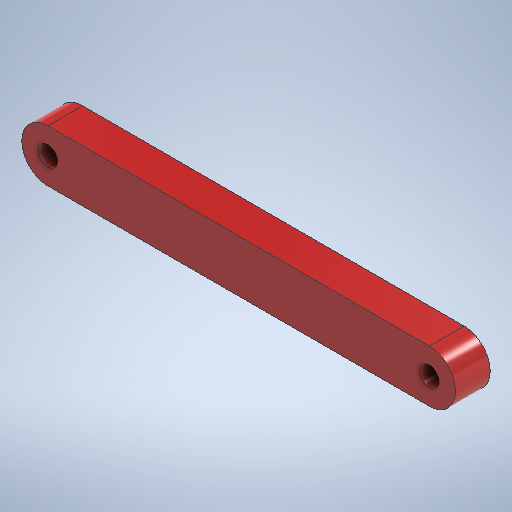
# Autodesk Inventor part: servostrap
Saved by Autodesk Inventor 2025.2 (Build 292293000, 293)
## iProperties
Created: 2025-04-02
Part Number: servostrap
Material: Generic
Document SubType Name: Modeling
Designer: m_kni
Density: 1 g/cm^3
Appearance: Default
Author: m_kni
## iProperties of the stored document servostrap_3DPrint.ipt
Created: 2025-04-02
Part Number: servostrap_3DPrint
Material: Generic
Document SubType Name: Modeling
Designer: m_kni
Density: 1 g/cm^3
Appearance: Default
Author: m_kni
Autodesk Inventor part; units mm, degrees
ref_plane "YZ Plane" through (0, 0, 0) normal (1, 0, 0) x (0, 1, 0)
ref_plane "XZ Plane" through (0, 0, 0) normal (0, 1, 0) x (-1, 0, 0)
ref_plane "XY Plane" through (0, 0, 0) normal (0, 0, 1) x (1, 0, 0)
sketch "Sketch1" plane through (0, 0, 0) normal (0, 0, 1) x (1, 0, 0)
  circle A0 centre (-21.9525, -0.0633) radius 1
  circle A1 centre (22.0475, -0.0633) radius 1
  circle A2 centre (-21.9525, -0.0633) radius 1.125
  circle A3 centre (22.0475, -0.0633) radius 1.125
  circle A4 centre (-21.9525, -0.0633) radius 3
  circle A5 centre (22.0475, -0.0633) radius 3
  line L0 (-21.9525, 2.9367) -> (22.0475, 2.9367)
  line L1 (-21.9525, -3.0633) -> (22.0475, -3.0633)
  point P0 (0, 0)
  dimension "d0" = 2.25
  dimension "d1" = 2.25
  dimension "d2" = 6
  dimension "d3" = 6
  constraints: 6 centre point, 4 coincident, 4 end point, 4 point on circle, 2 tangent
  measures "d0" diameter of A2
  measures "d1" diameter of A3
  measures "d2" diameter of A4
  measures "d3" diameter of A5
extrude "Extrusion1" add sketch "Sketch1" along normal blind 4 contours A4 | A4 L0 A5 L1 | A5
body "Solid1"
